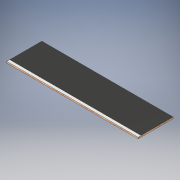
# Autodesk Inventor part: floorTopLayer
Saved by Autodesk Inventor 2017 (Build 210142000, 142)
## iProperties
Created: 2016-12-21
Part Number: floorTopLayer
Material: Wood (Birch)
Document SubType Name: Modeling
Designer: Naga
Density: 0.55 g/cm^3
Appearance: Birch - Natural Polished
Author: Naga
Autodesk Inventor part; units mm, degrees
ref_plane "YZ Plane" through (0, 0, 0) normal (1, 0, 0) x (0, 1, 0)
ref_plane "XZ Plane" through (0, 0, 0) normal (0, 1, 0) x (-1, 0, 0)
ref_plane "XY Plane" through (0, 0, 0) normal (0, 0, 1) x (1, 0, 0)
sketch "Sketch1" plane through (0, 0, 0) normal (0, 1, 0) x (-1, 0, 0)
  line L0 (-571.5, 152.4) -> (571.5, 152.4)
  line L1 (571.5, 152.4) -> (571.5, -152.4)
  line L2 (571.5, -152.4) -> (-571.5, -152.4)
  line L3 (-571.5, -152.4) -> (-571.5, 152.4)
  line L4 (-571.5, 152.4) -> (571.5, -152.4) construction
  line L5 (571.5, 152.4) -> (-571.5, -152.4) construction
  point P0 (0, 0)
  dimension "d0" = 1143
  dimension "d1" = 304.8
  constraints: 12 end point, 2 midpoint, 2 parallel, 1 horizontal, 1 perpendicular
  measures "d0" distance of L1.end L2.end
  measures "d1" distance of L0.end L1.end
extrude "Extrusion1" add sketch "Sketch1" along normal blind 12.7
sketch "Sketch2" plane through (0, 12.7, 0) normal (0, 1, 0) x (1, 0, 0)
  line L0 (-571.5, -152.4) -> (571.5, -152.4) projected
  line L1 (571.5, -152.4) -> (571.5, 152.4) projected
  line L2 (-571.5, -152.4) -> (571.5, -152.4)
  line L3 (571.5, -152.4) -> (571.5, -127)
  line L4 (571.5, -127) -> (-571.5, -127)
  line L5 (-571.5, -127) -> (-571.5, -152.4)
  point P0 (0, 0)
  dimension "d4" = 25.4
  constraints: 8 end point, 2 parallel, 1 horizontal, 1 perpendicular, 1 point on line
  measures "d4" distance of L3.end L2.end
extrude "Extrusion2" cut sketch "Sketch2" against normal blind 0.0254
body "Solid1"
